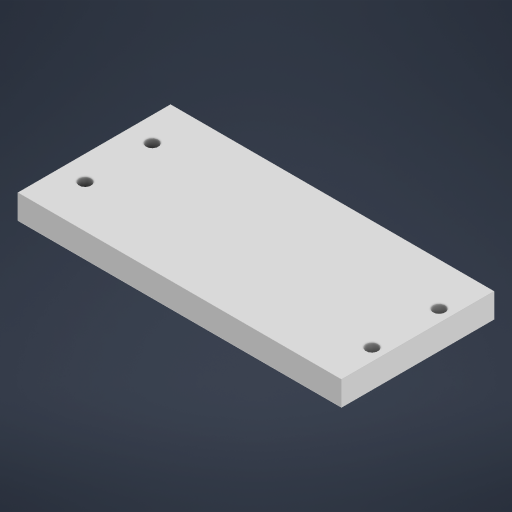
# Autodesk Inventor part: Langbektang houder
Saved by Autodesk Inventor 2023.2 (Build 272271000, 271)
## iProperties
Created: 2020-09-09
Part Number: Langbektang houder
Material: Generic
Document SubType Name: Modeling
Designer: nathan.bollaert
Density: 1 g/cm^3
Appearance: Default
Author: nathan.bollaert
Autodesk Inventor part; units mm, degrees
ref_plane "YZ Plane" through (0, 0, 0) normal (1, 0, 0) x (0, 1, 0)
ref_plane "XZ Plane" through (0, 0, 0) normal (0, 1, 0) x (-1, 0, 0)
ref_plane "XY Plane" through (0, 0, 0) normal (0, 0, 1) x (1, 0, 0)
sketch "Sketch1" plane through (0, 0, 0) normal (0, 1, 0) x (-1, 0, 0)
  line L0 (0, 0) -> (53, 0)
  line L1 (53, 0) -> (53, -25)
  line L2 (53, -25) -> (0, -25)
  line L3 (0, -25) -> (0, 0)
  circle A0 centre (49, -18) radius 1
  circle A1 centre (49, -7) radius 1
  line L4 (53, -12.5) -> (0, -12.5)
  line L5 (26.5, 0) -> (26.5, -25)
  circle A2 centre (2, -18) radius 1
  circle A3 centre (2, -7) radius 1
  dimension "d228" = 25
  dimension "d229" = 53
  dimension "d232" = 11
  dimension "d233" = 4
  dimension "d234" = 2
  dimension "d240" = 2
  constraints: 12 end point, 4 centre point, 4 midpoint, 2 parallel, 2 vertical alignment, 1 equal radius, 1 horizontal, 1 horizontal alignment, 1 perpendicular, 2 other
  measures "d228" distance of L0.end L1.end
  measures "d229" distance of L1.end L2.end
  measures "d232" distance of A0.centre A1.centre
  measures "d233" distance from line of L1 A0.centre
  measures "d234" diameter of A0
  measures "d240" distance from line of L3 A2.centre
extrude "Extrusion1" add sketch "Sketch1" against normal blind 4
body "Solid5"
